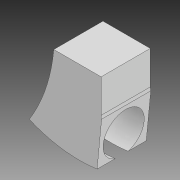
# Autodesk Inventor part: ORingToolA
Saved by Autodesk Inventor 2020 (Build 240168000, 168)
## iProperties
Created: 2020-12-25
Part Number: ORingToolA
Material: Generic
Document SubType Name: Modeling
Designer: DDeGo
Density: 1 g/cm^3
Appearance: Default
Author: DDeGo
Autodesk Inventor part; units mm, degrees
ref_plane "YZ Plane" through (0, 0, 0) normal (1, 0, 0) x (0, 1, 0)
ref_plane "XZ Plane" through (0, 0, 0) normal (0, 1, 0) x (-1, 0, 0)
sketch "Block1" plane through (0, 0, 0) normal (0, 0, 1) x (1, 0, 0)
  arc A0 (19.4993, -13.8282) -> (19.4817, -14.1291) centre (20.4774, -14.0361) ccw construction
  line L0 (19.4993, -13.8282) -> (20.7824, -7.7917) construction
  arc A1 (21.6494, -6.5302) -> (20.7824, -7.7917) centre (22.7387, -8.2075) ccw construction
  line L1 (21.6494, -6.5302) -> (21.8911, -6.3732) construction
  arc A2 (21.8911, -6.3732) -> (16.2026, -4.7141) centre (18.9149, -5.9962) ccw construction
  arc A3 (16.1932, -4.631) -> (16.2026, -4.7141) centre (16.693, -4.6165) ccw construction
  arc A4 (16.2, -5.1) -> (16.1932, -4.631) centre (0, -5.1) ccw construction
  arc A5 (11.587, -16.123) -> (16.2, -5.1) centre (0, -4.7972) ccw construction
  arc A6 (11.587, -16.123) -> (18.1044, -18.4699) centre (18.9149, -5.9962) ccw construction
  line L2 (19.4817, -14.1291) -> (18.1044, -18.4699) construction
  circle A7 centre (18.9149, -5.9962) radius 1 construction
  arc A8 (21.7954, -6.3313) -> (16.3027, -4.7365) centre (18.9149, -5.9962) ccw
  arc A9 (21.7954, -6.3313) -> (20.6845, -7.7709) centre (22.7387, -8.2075) ccw
  line L3 (20.6845, -7.7709) -> (19.4014, -13.8074)
  arc A10 (19.4014, -13.8074) -> (19.3804, -14.1177) centre (20.4774, -14.0361) ccw
  line L4 (19.3804, -14.1177) -> (18.0329, -18.3647)
  arc A11 (11.7396, -16.1093) -> (18.0329, -18.3647) centre (18.9149, -5.9962) ccw
  arc A12 (11.7396, -16.1093) -> (16.3027, -4.7365) centre (0, -4.7972) ccw
  line L5 (15.5605, -9.6605) -> (20.0788, -10.6209)
  point P0 (17.4447, -9.0721)
  dimension "d0" = 0.1
  dimension "d1" = 8
  measures "d0" radial gap between concentric circles of A12 A5
  measures "d1" distance from line of L4.end L5
sketch "Sketch1" plane through (0, 0, 0) normal (0, 0, 1) x (1, 0, 0)
  circle A0 centre (0, 0) radius 10.5 construction
  line L0 (-5.5192, -8.9325) -> (1.2791, -13.1329) construction
  arc A1 (2.2, -7.5394) -> (2.2454, -7.8373) centre (3.2, -7.5394) ccw construction
  line L1 (2.2, -7.5394) -> (2.2, -1.368) construction
  arc A2 (2.7858, 0.0462) -> (2.2, -1.368) centre (4.2, -1.368) ccw construction
  line L2 (2.7858, 0.0462) -> (2.9896, 0.25) construction
  arc A3 (2.9896, 0.25) -> (-2.9195, 0.6901) centre (0, 0) ccw construction
  arc A4 (-2.946, 0.7695) -> (-2.9195, 0.6901) centre (-2.4602, 0.8876) ccw construction
  arc A5 (-2.8419, 0.3121) -> (-2.946, 0.7695) centre (-18.6879, -3.0561) ccw construction
  arc A6 (-5.0623, -11.4291) -> (-2.8419, 0.3121) centre (-18.7508, -2.7598) ccw construction
  arc A7 (-5.0623, -11.4291) -> (1.8007, -12.3696) centre (0, 0) ccw construction
  line L3 (2.2454, -7.8373) -> (1.8007, -12.3696) construction
  circle A8 centre (0, 0) radius 1 construction
  arc A9 (2.8873, 0.2711) -> (-2.817, 0.689) centre (0, 0) ccw
  arc A10 (2.8873, 0.2711) -> (2.1, -1.368) centre (4.2, -1.368) ccw
  line L4 (2.1, -1.368) -> (2.1, -7.5394)
  arc A11 (2.1, -7.5394) -> (2.144, -7.8473) centre (3.2, -7.5394) ccw
  line L5 (2.144, -7.8473) -> (1.7089, -12.2817)
  arc A12 (-4.9158, -11.384) -> (1.7089, -12.2817) centre (0, 0) ccw
  arc A13 (-4.9158, -11.384) -> (-2.817, 0.689) centre (-18.7508, -2.7598) ccw
  line L6 (-2.5192, -4.2817) -> (2.1, -4.2817)
  dimension "d4" = 21
  dimension "d5" = 3
  constraints: 2 end point, 1 coincident, 5 other
extrude "Extrusion1" add sketch "Sketch1" along normal mid plane 4.8 contours L6 L4 A11 L5 A12 A13
ref_plane "Work Plane1" through (-5.5192, -8.9325, 0) normal (0.85071, -0.5256353, 0) x (0.5256353, 0.85071, 0)
sketch "Sketch2" plane through (-5.5192, -8.9325, 0) normal (0.85071, -0.5256353, 0) x (0.5256353, 0.85071, 0)
  circle A0 centre (0, 0) radius 2
  line L0 (10.5, -2.8) -> (10.5, 2.8) projected
  point P0 (10.5, 0)
  dimension "d6" = 4
  constraints: 1 centre point, 1 coincident
  measures "d6" diameter of A0
revolve "Revolution1" cut sketch "Sketch2" angle 360 about axis through (0, 0, 0) along (0, 0, 1)
body "Solid1"
